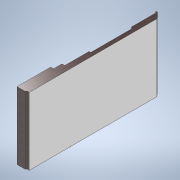
# Autodesk Inventor part: BlueShip-ver1-1111-2021
Saved by Autodesk Inventor 2021 (Build 250183000, 183)
## iProperties
Created: 2021-02-04
Part Number: BlueShip-ver1-1111-2021
Material: Wood (Oak)
Document SubType Name: Modeling
Designer: CMurray
Density: 0.76 g/cm^3
Appearance: Machined - Aluminum
Author: CMurray
Autodesk Inventor part; units mm, degrees
ref_plane "YZ Plane" through (0, 0, 0) normal (1, 0, 0) x (0, 1, 0)
ref_plane "XZ Plane" through (0, 0, 0) normal (0, 1, 0) x (-1, 0, 0)
sketch "Sketch1" plane through (0, 0, 0) normal (0, 1, 0) x (-1, 0, 0)
  line L0 (0, 0) -> (1023.9919, 0)
  line L1 (1023.9919, 0) -> (1023.9919, -167.3096)
  line L2 (0, 0) -> (508, 0)
  line L3 (1023.9919, 0) -> (660.4, 0)
  line L4 (660.4, 0) -> (611.4196, -58.3726)
  arc A0 (611.4196, -58.3726) -> (-38.1005, -58.3726) centre (286.6596, -2124.0484) ccw
  line L5 (1023.9919, 0) -> (660.4, 0)
  line L6 (769.9919, -1524) -> (769.9919, -6090.706)
  arc A1 (-38.1005, -4189.7242) -> (769.9919, -6090.706) centre (2601.9104, -4189.7242) ccw
  line L7 (-38.1005, -58.3726) -> (-38.1005, -4189.7242)
  line L8 (1023.9919, 0) -> (1023.9919, -1524)
  line L9 (1023.9919, -1524) -> (769.9919, -1524)
  dimension "d1" = 6096
  dimension "d2" = 508
  dimension "d11" = 76.2
  dimension "d12" = 130
  dimension "d49" = 1524
  dimension "d51" = 254
  constraints: 20 end point, 6 point on circle, 3 perpendicular, 2 centre point, 2 point on line, 1 collinear, 1 horizontal, 1 tangent, 1 vertical
  measures "d1" distance of L0.end L6.end
  measures "d2" distance of L0.start L2.end
  measures "d11" distance of L3.end L4.end
  measures "d12" angle of L0 L4
  measures "d49" distance of L0.end L8.end
  measures "d51" distance between parallel lines of L6 L8
extrude "Extrusion1" add sketch "Sketch1" along normal blind 3048
sketch "Sketch6" plane through (-769.9919, 0, -6090.706) normal (-1, 0, 0) x (0, 0, 1)
  line L0 (0, 0) -> (0, 3048) projected
  line L1 (0, 0) -> (4566.706, 0) projected
  line L2 (0, 3048) -> (50.8, 3048)
  line L3 (50.8, 3048) -> (50.8, 0)
  line L4 (50.8, 0) -> (0, 0)
  line L5 (0, 0) -> (0, 3048)
  point P0 (6090.706, 0)
  dimension "d33" = 50.8
  constraints: 8 end point, 2 parallel, 1 horizontal, 1 perpendicular, 1 point on line
  measures "d33" distance between parallel lines of L3 L0
extrude "Extrusion6" add sketch "Sketch6" along normal blind 50.8
fillet "Fillet1" radius 25.4 1 edges at (-820.7919, 1524, -6039.906)
fillet "Fillet2" radius 6.35 1 edges at (-820.7919, 1524, -6090.706)
fillet "Fillet4" radius 25.4 1 edges at (38.1005, 1524, -58.3726)
fillet "Fillet7" radius 6.35 1 edges at (-1023.9919, 1524, 0)
sketch "Sketch11" plane through (-769.9919, 0, -1524) normal (-1, 0, 0) x (0, 0, 1)
  line L0 (0, 0) -> (0, 3048) projected
  line L1 (-4515.906, 0) -> (0, 0) projected
  line L2 (0, 3048) -> (-4515.906, 3048)
  line L3 (-4515.906, 3048) -> (-4515.906, 0)
  line L4 (-4515.906, 0) -> (0, 0)
  line L5 (0, 0) -> (0, 3048)
  line L6 (-4515.906, 0) -> (0, 0)
  line L7 (0, 0) -> (0, 3048)
  line L8 (0, 3048) -> (-4515.906, 3048)
  line L9 (-4515.906, 3048) -> (-4515.906, 0)
  line L10 (-50.8, 2997.2) -> (-3727.5531, 2997.2)
  line L11 (-3727.5531, 50.8) -> (-50.8, 50.8)
  line L12 (-50.8, 50.8) -> (0, 50.8)
  line L13 (-50.8, 2997.2) -> (0, 2997.2)
  line L14 (-3727.5531, 50.8) -> (-4235.5531, 50.8)
  line L15 (-4235.5531, 50.8) -> (-4489.5531, 50.8)
  line L16 (-4489.5531, 50.8) -> (-4489.5531, 2997.2)
  line L17 (-4489.5531, 2997.2) -> (-3727.5531, 2997.2)
  point P0 (1524, 0)
  dimension "d55" = 50.8
  dimension "d56" = 50.8
  dimension "d94" = 508
  dimension "d95" = 254
  constraints: 32 end point, 5 perpendicular, 4 parallel, 3 horizontal, 3 point on line, 1 collinear
  measures "d55" distance between parallel lines of L2 L10
  measures "d56" distance between parallel lines of L1 L11
  measures "d94" distance of L11.start L14.end
  measures "d95" distance of L14.end L15.end
extrude "Extrusion9" cut sketch "Sketch11" against normal blind 76.2 contours L12 L11 L14 L15 L16 L17 L10 L13 L0
ref_plane "Work Plane12" through (-515.9919, 0, -1905) normal (-1, 0, 0) x (0, 0, 1)
sketch "Sketch12" plane through (-515.9919, 0, -1905) normal (-1, 0, 0) x (0, 0, 1)
  line L0 (2216.3698, -160.707) -> (-4488.1257, -160.707)
  line L1 (-4488.1257, -160.707) -> (-4488.1257, 3204.096)
  line L2 (-4488.1257, 3204.096) -> (2216.3698, 3204.096)
  line L3 (2216.3698, 3204.096) -> (2216.3698, -160.707)
  point P0 (1905, 0)
  constraints: 8 end point, 2 parallel, 1 horizontal, 1 perpendicular
extrude "Extrusion10" cut sketch "Sketch12" against normal blind 1270
ref_plane "Work Plane13" through (-515.9919, 3048, -3043.1155) normal (1, 0, 0) x (0, 0, -1)
sketch "Sketch13" plane through (0, 3048, 0) normal (0, 1, 0) x (1, 0, 0)
  line L0 (-769.9919, 6039.906) -> (-769.9919, 1524) projected
  line L1 (-769.9919, 1524) -> (-769.9919, 3004.9849)
  line L2 (-769.9919, 6039.9575) -> (-769.9919, 4896.9575)
  line L3 (-769.9919, 3004.9849) -> (-693.7919, 3004.9849)
  line L4 (-693.7919, 3004.9849) -> (-693.7919, 4896.9575)
  line L5 (-693.7919, 6013.5531) -> (-693.7919, 1524) projected
  line L6 (-769.9919, 4896.9575) -> (-693.7919, 4896.9575)
  point P0 (0, 0)
  point P1 (-693.7919, 5251.5531)
  point P2 (-693.7919, 6014.208)
  dimension "d62" = 1143
  dimension "d63" = 76.2
  constraints: 10 end point, 4 point on line, 1 horizontal, 1 perpendicular
  measures "d62" distance of L2.start L2.end
  measures "d63" distance of L1.end L3.end
extrude "Extrusion11" cut sketch "Sketch13" against normal blind 1524
fillet "Fillet8" radius 25.4 1 edges at (-769.9919, 3022.6, -3004.9849)
fillet "Fillet10" radius 25.4 1 edges at (-769.9919, 3022.6, -4896.9575)
sketch "Sketch16" plane through (-769.9919, 2997.2, -1524) normal (-1, 0, 0) x (0, 0, 1)
  line L0 (0, 50.8) -> (-718.9849, 50.8)
  line L1 (-718.9849, 50.8) -> (-718.9849, 203.1957)
  line L2 (-1455.5849, 50.8) -> (0, 50.8) projected
  line L3 (-1480.9849, 0) -> (0, 0) projected
  line L4 (0, 50.8) -> (-1480.9849, 50.8)
  line L5 (-1480.9849, 50.8) -> (-1480.9849, 0)
  line L6 (-1480.9849, 0) -> (0, 0)
  line L7 (0, 0) -> (0, 50.8)
  line L8 (0, 50.8) -> (-381, 50.8)
  line L9 (-381, 50.8) -> (-381, 0)
  line L10 (-381, 0) -> (0, 0)
  line L11 (0, 0) -> (0, 50.8)
  point P0 (1524, -2997.2)
  point P1 (-381, 50.8)
  point P2 (-381, 0)
  point P3 (0, 0)
  dimension "d78" = 381
  constraints: 20 end point, 4 parallel, 3 horizontal, 3 perpendicular, 1 point on line
  measures "d78" distance of L10.end L9.end
extrude "Extrusion14" add sketch "Sketch16" along normal blind 127 contours L7 L3 L9 L0
fillet "Fillet13" radius 25.4 1 edges at (-896.9919, 3022.6, -1905)
sketch "Sketch17" plane through (-769.9919, 0, -6039.906) normal (-1, 0, 0) x (0, 0, 1)
  line L0 (4515.906, 50.8) -> (26.3529, 50.8) projected
  line L1 (4515.906, 0) -> (4134.906, 0)
  line L2 (4134.906, 0) -> (4134.906, 50.8)
  line L3 (4134.906, 50.8) -> (4515.906, 50.8)
  line L4 (4515.906, 50.8) -> (4515.906, 0)
  point P0 (6039.906, 0)
  point P1 (25.698, 50.8)
  point P2 (788.3529, 50.8)
  dimension "d83" = 381
  constraints: 8 end point, 2 parallel, 1 horizontal, 1 perpendicular, 1 point on line
  measures "d83" distance of L2.end L3.end
extrude "Extrusion15" add sketch "Sketch17" along normal blind 127
fillet "Fillet15" radius 25.4 1 edges at (-896.9919, 25.4, -1905)
sketch "Sketch18" plane through (-1023.9919, 0, -1524) normal (-1, 0, 0) x (0, 0, 1)
  line L0 (0, 3048) -> (-355.6, 3048) projected
  line L1 (1524, 0) -> (0, 0)
  line L2 (0, 0) -> (0, 3048)
  line L3 (0, 3048) -> (1524, 3048)
  line L4 (1524, 3048) -> (1524, 0)
  line L5 (1473.2, 50.8) -> (50.8, 50.8)
  line L6 (50.8, 2997.2) -> (1473.2, 2997.2)
  line L7 (1473.2, 2997.2) -> (1473.2, 50.8)
  line L8 (50.8, 2997.2) -> (0, 2997.2)
  line L9 (0, 0) -> (0, 3048) projected
  line L10 (50.8, 50.8) -> (0, 50.8)
  point P0 (0, 2997.2)
  dimension "d88" = 50.8
  constraints: 18 end point, 4 parallel, 2 perpendicular, 2 point on line, 1 horizontal, 1 other
  measures "d88" distance between parallel lines of L4 L7
extrude "Extrusion16" cut sketch "Sketch18" against normal blind 76.2 contours L2 L8 L6 L7 L5 L10
fillet "Fillet17" radius 25.4 1 edges at (-1023.9919, 3022.6, -1524)
fillet "Fillet18" radius 25.4 1 edges at (-1023.9919, 25.4, -1524)
fillet "Fillet19" radius 38.1 1 edges at (-947.7919, 1524, -1524)
sketch "Sketch19" plane through (-947.7919, 0, -1524) normal (-1, 0, 0) x (0, 0, 1)
  line L0 (0, 2997.2) -> (38.1, 2997.2) projected
  line L1 (1473.2, 50.8) -> (38.1, 50.8)
  line L2 (38.1, 50.8) -> (38.1, 2997.2)
  line L3 (38.1, 2997.2) -> (1473.2, 2997.2)
  line L4 (1473.2, 2997.2) -> (1473.2, 50.8)
  line L5 (165.1, 2870.2) -> (165.1, 177.8)
  line L6 (165.1, 177.8) -> (1346.2, 177.8)
  line L7 (1346.2, 177.8) -> (1346.2, 2870.2)
  line L8 (1346.2, 2870.2) -> (165.1, 2870.2)
  point P0 (1524, 0)
  dimension "d96" = 127
  constraints: 16 end point, 4 parallel, 2 perpendicular, 1 horizontal, 3 other
  measures "d96" distance between parallel lines of L2 L5
extrude "Extrusion17" cut sketch "Sketch19" against normal blind 165.1 contours L8 L7 L6 L5
fillet "Fillet20" radius 25.4 1 edges at (-947.7919, 177.8, -768.35)
fillet "Fillet21" radius 25.4 2 edges at (-947.7919, 165.1, -177.8) (-947.7919, 1524, -177.8)
fillet "Fillet22" radius 25.4 2 edges at (-947.7919, 1524, -1358.9) (-947.7919, 165.1, -1358.9)
fillet "Fillet23" radius 25.4 3 edges at (-947.7919, 2870.2, -1371.6) (-947.7919, 2870.2, -768.35) (-947.7919, 2870.2, -165.1)
body "Solid1"
